Autodesk Fusion 360 part; units mm, degrees
note: some values were not read from the file. Set by a fixed rule: which sketch regions a step uses.
(part 2 of 10)
  spline S7 degree 5 poles (14.007, -3.8365) (14.007, -3.8365) (14.0072, -3.8366) (14.0074, -3.8366) (14.0077, -3.8367) (14.0083, -3.8369) (14.0089, -3.837) (14.0095, -3.8372) (14.0103, -3.8374) (14.0111, -3.8376) (14.012, -3.8378) (14.013, -3.838) (14.0141, -3.8383) (14.0152, -3.8386) (14.0164, -3.8388) (14.0177, -3.8391) (14.019, -3.8394) (14.0204, -3.8398) (14.0219, -3.8401) (14.0235, -3.8405) (14.0251, -3.8408) (14.0268, -3.8412) (14.0286, -3.8416) (14.0305, -3.842) (14.0324, -3.8424) (14.0343, -3.8428) (14.0364, -3.8432) (14.0385, -3.8436) (14.0407, -3.8441) (14.0429, -3.8445) (14.0452, -3.845) (14.0476, -3.8454) (14.05, -3.8459) (14.0525, -3.8464) (14.0551, -3.8469) (14.0577, -3.8473) (14.0604, -3.8478) (14.0632, -3.8483) (14.066, -3.8488) (14.0688, -3.8493) (14.0718, -3.8498) (14.0748, -3.8504) (14.0778, -3.8509) (14.0809, -3.8514) (14.0841, -3.8519) (14.0873, -3.8525) (14.0906, -3.853) (14.094, -3.8535) (14.0974, -3.854) (14.1009, -3.8546) (14.1044, -3.8551) (14.1079, -3.8557) (14.1116, -3.8562) (14.1153, -3.8567) (14.119, -3.8573) (14.1228, -3.8578) (14.1267, -3.8583) (14.1306, -3.8589) (14.1345, -3.8594) (14.1386, -3.86) (14.1426, -3.8605) (14.1467, -3.861) (14.1509, -3.8615) (14.1552, -3.8621) (14.1594, -3.8626) (14.1638, -3.8631) (14.1682, -3.8636) (14.1726, -3.8642) (14.1771, -3.8647) (14.1816, -3.8652) (14.1862, -3.8657) (14.1908, -3.8662) (14.1955, -3.8667) (14.2003, -3.8672) (14.2051, -3.8677) (14.2099, -3.8682) (14.2148, -3.8686) (14.2197, -3.8691) (14.2247, -3.8696) (14.2297, -3.87) (14.2348, -3.8705) (14.2399, -3.871) (14.2451, -3.8714) (14.2503, -3.8718) (14.2556, -3.8723) (14.2609, -3.8727) (14.2663, -3.8731) (14.2717, -3.8735) (14.2771, -3.8739) (14.2826, -3.8743) (14.2882, -3.8747) (14.2938, -3.8751) (14.2994, -3.8755) (14.3051, -3.8758) (14.3108, -3.8762) (14.3166, -3.8766) (14.3224, -3.8769) (14.3283, -3.8772) (14.3342, -3.8776) (14.3401, -3.8779) (14.3461, -3.8782) (14.3521, -3.8785) (14.3582, -3.8788) (14.3643, -3.879) (14.3705, -3.8793) (14.3767, -3.8796) (14.3829, -3.8798) (14.3892, -3.88) (14.3955, -3.8803) (14.4019, -3.8805) (14.4083, -3.8807) (14.4147, -3.8809) (14.4212, -3.8811) (14.4277, -3.8812) (14.4343, -3.8814) (14.4409, -3.8816) (14.4476, -3.8817) (14.4542, -3.8818) (14.461, -3.8819) (14.4677, -3.882) (14.4745, -3.8821) (14.4814, -3.8822) (14.4883, -3.8823) (14.4952, -3.8823) (14.5021, -3.8824) (14.5091, -3.8824) (14.5162, -3.8824) (14.5233, -3.8824) (14.5304, -3.8824) (14.5375, -3.8824) (14.5447, -3.8824) (14.5519, -3.8823) (14.5592, -3.8823) (14.5665, -3.8822) (14.5738, -3.8821) (14.5812, -3.882) (14.5886, -3.8819) (14.596, -3.8817) (14.6035, -3.8816) (14.611, -3.8814) (14.6186, -3.8813) (14.6261, -3.8811) (14.6338, -3.8809) (14.6414, -3.8807) (14.6491, -3.8804) (14.6568, -3.8802) (14.6646, -3.8799) (14.6724, -3.8797) (14.6802, -3.8794) (14.6881, -3.8791) (14.696, -3.8787) (14.7039, -3.8784) (14.7119, -3.878) (14.7199, -3.8777) (14.7279, -3.8773) (14.7359, -3.8769) (14.744, -3.8765) (14.7522, -3.8761) (14.7603, -3.8756) (14.7685, -3.8751) (14.7768, -3.8747) (14.785, -3.8742) (14.7933, -3.8737) (14.8016, -3.8731) (14.81, -3.8726) (14.8184, -3.872) (14.8268, -3.8714) (14.8352, -3.8708) (14.8437, -3.8702) (14.8522, -3.8696) (14.8608, -3.869) (14.8693, -3.8683) (14.8779, -3.8676) (14.8866, -3.8669) (14.8952, -3.8662) (14.9039, -3.8655) (14.9127, -3.8647) (14.9214, -3.8639) (14.9302, -3.8632) (14.939, -3.8624) (14.9479, -3.8615) (14.9567, -3.8607) (14.9656, -3.8598) (14.9746, -3.859) (14.9835, -3.8581) (14.9925, -3.8572) (15.0015, -3.8562) (15.0106, -3.8553) (15.0197, -3.8543) (15.0288, -3.8533) (15.0379, -3.8523) (15.0471, -3.8513) (15.0563, -3.8503) (15.0655, -3.8492) (15.0747, -3.8481) (15.084, -3.847) (15.0933, -3.8459) (15.1026, -3.8448) (15.112, -3.8436) (15.1214, -3.8424) (15.1308, -3.8412) (15.1402, -3.84) (15.1497, -3.8388) (15.1591, -3.8375) (15.1687, -3.8363) (15.1782, -3.835) (15.1878, -3.8337) (15.1974, -3.8323) (15.207, -3.831) (15.2166, -3.8296) (15.2263, -3.8282) (15.236, -3.8268) (15.2457, -3.8254) (15.2555, -3.8239) (15.2653, -3.8225) (15.2751, -3.821) (15.2849, -3.8195) (15.2947, -3.8179) (15.3046, -3.8164) (15.3145, -3.8148) (15.3244, -3.8132) (15.3344, -3.8116) (15.3444, -3.81) (15.3544, -3.8083) (15.3644, -3.8067) (15.3744, -3.805) (15.3845, -3.8033) (15.3946, -3.8015) (15.4047, -3.7998) (15.4148, -3.798) (15.425, -3.7962) (15.4352, -3.7944) (15.4454, -3.7925) (15.4556, -3.7907) (15.4659, -3.7888) (15.4762, -3.7869) (15.4865, -3.7849) (15.4968, -3.783) (15.5072, -3.781) (15.5175, -3.779) (15.5279, -3.777) (15.5363, -3.7754) (15.5425, -3.7742) (15.5467, -3.7733) (15.5488, -3.7729) knots 0 0 0 0 0 0 0.00416667 0.00833333 0.0125 0.01666667 0.02083333 0.025 0.02916667 0.03333333 0.0375 0.04166667 0.04583333 0.05 0.05416667 0.05833333 0.0625 0.06666667 0.07083333 0.075 0.07916667 0.08333333 0.0875 0.09166667 0.09583333 0.1 0.10416667 0.10833333 0.1125 0.11666667 0.12083333 0.125 0.12916667 0.13333333 0.1375 0.14166667 0.14583333 0.15 0.15416667 0.15833333 0.1625 0.16666667 0.17083333 0.175 0.17916667 0.18333333 0.1875 0.19166667 0.19583333 0.2 0.20416667 0.20833333 0.2125 0.21666667 0.22083333 0.225 0.22916667 0.23333333 0.2375 0.24166667 0.24583333 0.25 0.25416667 0.25833333 0.2625 0.26666667 0.27083333 0.275 0.27916667 0.28333333 0.2875 0.29166667 0.29583333 0.3 0.30416667 0.30833333 0.3125 0.31666667 0.32083333 0.325 0.32916667 0.33333333 0.3375 0.34166667 0.34583333 0.35 0.35416667 0.35833333 0.3625 0.36666667 0.37083333 0.375 0.37916667 0.38333333 0.3875 0.39166667 0.39583333 0.4 0.40416667 0.40833333 0.4125 0.41666667 0.42083333 0.425 0.42916667 0.43333333 0.4375 0.44166667 0.44583333 0.45 0.45416667 0.45833333 0.4625 0.46666667 0.47083333 0.475 0.47916667 0.48333333 0.4875 0.49166667 0.49583333 0.5 0.50416667 0.50833333 0.5125 0.51666667 0.52083333 0.525 0.52916667 0.53333333 0.5375 0.54166667 0.54583333 0.55 0.55416667 0.55833333 0.5625 0.56666667 0.57083333 0.575 0.57916667 0.58333333 0.5875 0.59166667 0.59583333 0.6 0.60416667 0.60833333 0.6125 0.61666667 0.62083333 0.625 0.62916667 0.63333333 0.6375 0.64166667 0.64583333 0.65 0.65416667 0.65833333 0.6625 0.66666667 0.67083333 0.675 0.67916667 0.68333333 0.6875 0.69166667 0.69583333 0.7 0.70416667 0.70833333 0.7125 0.71666667 0.72083333 0.725 0.72916667 0.73333333 0.7375 0.74166667 0.74583333 0.75 0.75416667 0.75833333 0.7625 0.76666667 0.77083333 0.775 0.77916667 0.78333333 0.7875 0.79166667 0.79583333 0.8 0.80416667 0.80833333 0.8125 0.81666667 0.82083333 0.825 0.82916667 0.83333333 0.8375 0.84166667 0.84583333 0.85 0.85416667 0.85833333 0.8625 0.86666667 0.87083333 0.875 0.87916667 0.88333333 0.8875 0.89166667 0.89583333 0.9 0.90416667 0.90833333 0.9125 0.91666667 0.92083333 0.925 0.92916667 0.93333333 0.9375 0.94166667 0.94583333 0.95 0.95416667 0.95833333 0.9625 0.96666667 0.97083333 0.975 0.97916667 0.98333333 0.9875 0.99166667 0.99583333 1 1 1 1 1 1
  arc A6 (15.5488, -3.7729) -> (15.7391, -2.8775) centre (0, 0) ccw
  line L7 (12.9032, 6.6649) -> (12.9026, 6.6646)
  line L8 (13.5863, 5.129) -> (13.5869, 5.1293)
  arc A7 (14.7969, 6.087) -> (14.4246, 6.9233) centre (0, 0) ccw
  arc A8 (15.7391, 2.8775) -> (15.5488, 3.7729) centre (0, 0) ccw
  line L9 (12.8639, 4.8563) -> (13.5863, 5.129)
  circle A9 centre (-7.0711, -7.0711) radius 1.7
  spline S8 degree 5 poles (14.4985, -0.8405) (14.4986, -0.8405) (14.4987, -0.8405) (14.499, -0.8405) (14.4993, -0.8405) (14.4999, -0.8405) (14.5005, -0.8406) (14.5012, -0.8406) (14.502, -0.8406) (14.5028, -0.8406) (14.5037, -0.8407) (14.5048, -0.8407) (14.5058, -0.8407) (14.507, -0.8407) (14.5082, -0.8408) (14.5096, -0.8408) (14.5109, -0.8408) (14.5124, -0.8408) (14.5139, -0.8409) (14.5155, -0.8409) (14.5172, -0.8409) (14.519, -0.8409) (14.5208, -0.8409) (14.5226, -0.8409) (14.5246, -0.8409) (14.5266, -0.8409) (14.5287, -0.8409) (14.5309, -0.8409) (14.5331, -0.8408) (14.5354, -0.8408) (14.5377, -0.8408) (14.5401, -0.8407) (14.5426, -0.8407) (14.5452, -0.8406) (14.5478, -0.8406) (14.5504, -0.8405) (14.5532, -0.8404) (14.556, -0.8403) (14.5588, -0.8402) (14.5617, -0.8401) (14.5647, -0.84) (14.5677, -0.8399) (14.5708, -0.8398) (14.574, -0.8396) (14.5772, -0.8395) (14.5805, -0.8393) (14.5838, -0.8392) (14.5872, -0.839) (14.5906, -0.8388) (14.5941, -0.8386) (14.5977, -0.8384) (14.6013, -0.8382) (14.605, -0.838) (14.6087, -0.8377) (14.6124, -0.8375) (14.6163, -0.8372) (14.6202, -0.8369) (14.6241, -0.8366) (14.6281, -0.8363) (14.6321, -0.836) (14.6362, -0.8357) (14.6404, -0.8354) (14.6446, -0.835) (14.6488, -0.8347) (14.6531, -0.8343) (14.6574, -0.8339) (14.6618, -0.8335) (14.6663, -0.8331) (14.6708, -0.8326) (14.6753, -0.8322) (14.6799, -0.8317) (14.6846, -0.8313) (14.6893, -0.8308) (14.694, -0.8303) (14.6988, -0.8298) (14.7036, -0.8292) (14.7085, -0.8287) (14.7134, -0.8281) (14.7184, -0.8275) (14.7234, -0.8269) (14.7285, -0.8263) (14.7336, -0.8257) (14.7387, -0.8251) (14.7439, -0.8244) (14.7492, -0.8237) (14.7545, -0.8231) (14.7598, -0.8224) (14.7652, -0.8216) (14.7706, -0.8209) (14.7761, -0.8201) (14.7816, -0.8194) (14.7871, -0.8186) (14.7927, -0.8178) (14.7983, -0.817) (14.804, -0.8161) (14.8097, -0.8153) (14.8155, -0.8144) (14.8213, -0.8135) (14.8271, -0.8126) (14.833, -0.8117) (14.8389, -0.8107) (14.8449, -0.8097) (14.8509, -0.8088) (14.8569, -0.8078) (14.863, -0.8067) (14.8691, -0.8057) (14.8753, -0.8047) (14.8814, -0.8036) (14.8877, -0.8025) (14.8939, -0.8014) (14.9003, -0.8002) (14.9066, -0.7991) (14.913, -0.7979) (14.9194, -0.7967) (14.9259, -0.7955) (14.9324, -0.7943) (14.9389, -0.7931) (14.9455, -0.7918) (14.9521, -0.7905) (14.9587, -0.7892) (14.9654, -0.7879) (14.9721, -0.7865) (14.9788, -0.7852) (14.9856, -0.7838) (14.9924, -0.7824) (14.9993, -0.781) (15.0062, -0.7795) (15.0131, -0.778) (15.02, -0.7766) (15.027, -0.775) (15.0341, -0.7735) (15.0411, -0.772) (15.0482, -0.7704) (15.0553, -0.7688) (15.0625, -0.7672) (15.0697, -0.7656) (15.0769, -0.7639) (15.0841, -0.7622) (15.0914, -0.7605) (15.0987, -0.7588) (15.1061, -0.7571) (15.1135, -0.7553) (15.1209, -0.7535) (15.1283, -0.7517) (15.1358, -0.7499) (15.1433, -0.7481) (15.1508, -0.7462) (15.1584, -0.7443) (15.166, -0.7424) (15.1736, -0.7405) (15.1813, -0.7385) (15.1889, -0.7365) (15.1967, -0.7345) (15.2044, -0.7325) (15.2122, -0.7305) (15.22, -0.7284) (15.2278, -0.7263) (15.2357, -0.7242) (15.2436, -0.7221) (15.2515, -0.7199) (15.2594, -0.7177) (15.2674, -0.7155) (15.2754, -0.7133) (15.2834, -0.7111) (15.2915, -0.7088) (15.2996, -0.7065) (15.3077, -0.7042) (15.3158, -0.7018) (15.324, -0.6995) (15.3322, -0.6971) (15.3404, -0.6947) (15.3487, -0.6923) (15.3569, -0.6898) (15.3652, -0.6873) (15.3736, -0.6848) (15.3819, -0.6823) (15.3903, -0.6797) (15.3987, -0.6772) (15.4071, -0.6746) (15.4156, -0.672) (15.4241, -0.6693) (15.4326, -0.6667) (15.4411, -0.664) (15.4497, -0.6613) (15.4582, -0.6585) (15.4668, -0.6558) (15.4755, -0.653) (15.4841, -0.6502) (15.4928, -0.6473) (15.5015, -0.6445) (15.5102, -0.6416) (15.519, -0.6387) (15.5278, -0.6358) (15.5365, -0.6328) (15.5454, -0.6298) (15.5542, -0.6268) (15.5631, -0.6238) (15.572, -0.6207) (15.5809, -0.6177) (15.5898, -0.6146) (15.5988, -0.6114) (15.6077, -0.6083) (15.6167, -0.6051) (15.6258, -0.6019) (15.6348, -0.5987) (15.6439, -0.5955) (15.653, -0.5922) (15.6621, -0.5889) (15.6712, -0.5856) (15.6803, -0.5822) (15.6895, -0.5789) (15.6987, -0.5755) (15.7079, -0.572) (15.7172, -0.5686) (15.7264, -0.5651) (15.7357, -0.5616) (15.745, -0.5581) (15.7543, -0.5546) (15.7636, -0.551) (15.773, -0.5474) (15.7824, -0.5438) (15.7918, -0.5401) (15.8012, -0.5365) (15.8106, -0.5328) (15.8201, -0.529) (15.8295, -0.5253) (15.839, -0.5215) (15.8486, -0.5177) (15.8581, -0.5139) (15.8676, -0.5101) (15.8772, -0.5062) (15.8868, -0.5023) (15.8964, -0.4984) (15.906, -0.4944) (15.9157, -0.4904) (15.9253, -0.4864) (15.935, -0.4824) (15.9447, -0.4784) (15.9544, -0.4743) (15.9641, -0.4702) (15.9739, -0.466) (15.9817, -0.4627) (15.9876, -0.4602) (15.9915, -0.4585) (15.9935, -0.4577) knots 0 0 0 0 0 0 0.00416667 0.00833333 0.0125 0.01666667 0.02083333 0.025 0.02916667 0.03333333 0.0375 0.04166667 0.04583333 0.05 0.05416667 0.05833333 0.0625 0.06666667 0.07083333 0.075 0.07916667 0.08333333 0.0875 0.09166667 0.09583333 0.1 0.10416667 0.10833333 0.1125 0.11666667 0.12083333 0.125 0.12916667 0.13333333 0.1375 0.14166667 0.14583333 0.15 0.15416667 0.15833333 0.1625 0.16666667 0.17083333 0.175 0.17916667 0.18333333 0.1875 0.19166667 0.19583333 0.2 0.20416667 0.20833333 0.2125 0.21666667 0.22083333 0.225 0.22916667 0.23333333 0.2375 0.24166667 0.24583333 0.25 0.25416667 0.25833333 0.2625 0.26666667 0.27083333 0.275 0.27916667 0.28333333 0.2875 0.29166667 0.29583333 0.3 0.30416667 0.30833333 0.3125 0.31666667 0.32083333 0.325 0.32916667 0.33333333 0.3375 0.34166667 0.34583333 0.35 0.35416667 0.35833333 0.3625 0.36666667 0.37083333 0.375 0.37916667 0.38333333 0.3875 0.39166667 0.39583333 0.4 0.40416667 0.40833333 0.4125 0.41666667 0.42083333 0.425 0.42916667 0.43333333 0.4375 0.44166667 0.44583333 0.45 0.45416667 0.45833333 0.4625 0.46666667 0.47083333 0.475 0.47916667 0.48333333 0.4875 0.49166667 0.49583333 0.5 0.50416667 0.50833333 0.5125 0.51666667 0.52083333 0.525 0.52916667 0.53333333 0.5375 0.54166667 0.54583333 0.55 0.55416667 0.55833333 0.5625 0.56666667 0.57083333 0.575 0.57916667 0.58333333 0.5875 0.59166667 0.59583333 0.6 0.60416667 0.60833333 0.6125 0.61666667 0.62083333 0.625 0.62916667 0.63333333 0.6375 0.64166667 0.64583333 0.65 0.65416667 0.65833333 0.6625 0.66666667 0.67083333 0.675 0.67916667 0.68333333 0.6875 0.69166667 0.69583333 0.7 0.70416667 0.70833333 0.7125 0.71666667 0.72083333 0.725 0.72916667 0.73333333 0.7375 0.74166667 0.74583333 0.75 0.75416667 0.75833333 0.7625 0.76666667 0.77083333 0.775 0.77916667 0.78333333 0.7875 0.79166667 0.79583333 0.8 0.80416667 0.80833333 0.8125 0.81666667 0.82083333 0.825 0.82916667 0.83333333 0.8375 0.84166667 0.84583333 0.85 0.85416667 0.85833333 0.8625 0.86666667 0.87083333 0.875 0.87916667 0.88333333 0.8875 0.89166667 0.89583333 0.9 0.90416667 0.90833333 0.9125 0.91666667 0.92083333 0.925 0.92916667 0.93333333 0.9375 0.94166667 0.94583333 0.95 0.95416667 0.95833333 0.9625 0.96666667 0.97083333 0.975 0.97916667 0.98333333 0.9875 0.99166667 0.99583333 1 1 1 1 1 1
  arc A10 (13.727, 0.7957) -> (13.5924, 2.0756) centre (0, 0) ccw
  arc A11 (15.9935, -0.4577) -> (15.9935, 0.4577) centre (0, 0) ccw
  spline S9 degree 5 poles (15.7391, -2.8775) (15.7374, -2.8763) (15.7339, -2.8738) (15.7287, -2.8702) (15.7217, -2.8653) (15.713, -2.8592) (15.7044, -2.8532) (15.6957, -2.8472) (15.6871, -2.8412) (15.6785, -2.8353) (15.6698, -2.8293) (15.6612, -2.8234) (15.6526, -2.8176) (15.6441, -2.8117) (15.6355, -2.8059) (15.6269, -2.8002) (15.6184, -2.7944) (15.6099, -2.7887) (15.6014, -2.783) (15.5929, -2.7773) (15.5844, -2.7717) (15.5759, -2.7661) (15.5674, -2.7605) (15.559, -2.755) (15.5505, -2.7494) (15.5421, -2.744) (15.5337, -2.7385) (15.5253, -2.7331) (15.517, -2.7277) (15.5086, -2.7223) (15.5002, -2.7169) (15.4919, -2.7116) (15.4836, -2.7063) (15.4753, -2.7011) (15.467, -2.6958) (15.4587, -2.6906) (15.4505, -2.6855) (15.4422, -2.6803) (15.434, -2.6752) (15.4258, -2.6701) (15.4176, -2.665) (15.4094, -2.66) (15.4013, -2.655) (15.3931, -2.65) (15.385, -2.6451) (15.3769, -2.6402) (15.3688, -2.6353) (15.3607, -2.6304) (15.3527, -2.6256) (15.3446, -2.6208) (15.3366, -2.616) (15.3286, -2.6113) (15.3206, -2.6065) (15.3126, -2.6019) (15.3047, -2.5972) (15.2968, -2.5926) (15.2888, -2.588) (15.2809, -2.5834) (15.2731, -2.5788) (15.2652, -2.5743) (15.2574, -2.5698) (15.2495, -2.5654) (15.2417, -2.5609) (15.2339, -2.5565) (15.2262, -2.5522) (15.2184, -2.5478) (15.2107, -2.5435) (15.203, -2.5392) (15.1953, -2.5349) (15.1876, -2.5307) (15.18, -2.5265) (15.1724, -2.5223) (15.1648, -2.5182) (15.1572, -2.514) (15.1496, -2.5099) (15.1421, -2.5059) (15.1346, -2.5018) (15.1271, -2.4978) (15.1196, -2.4939) (15.1121, -2.4899) (15.1047, -2.486) (15.0973, -2.4821) (15.0899, -2.4782) (15.0825, -2.4744) (15.0752, -2.4706) (15.0679, -2.4668) (15.0606, -2.463) (15.0533, -2.4593) (15.0461, -2.4556) (15.0388, -2.4519) (15.0316, -2.4483) (15.0245, -2.4447) (15.0173, -2.4411) (15.0102, -2.4375) (15.0031, -2.434) (14.996, -2.4305) (14.9889, -2.427) (14.9819, -2.4236) (14.9749, -2.4201) (14.9679, -2.4167) (14.9609, -2.4134) (14.954, -2.41) (14.9471, -2.4067) (14.9402, -2.4034) (14.9334, -2.4002) (14.9266, -2.397) (14.9198, -2.3938) (14.913, -2.3906) (14.9062, -2.3874) (14.8995, -2.3843) (14.8928, -2.3812) (14.8862, -2.3782) (14.8795, -2.3751) (14.8729, -2.3721) (14.8663, -2.3691) (14.8598, -2.3662) (14.8533, -2.3633) (14.8468, -2.3604) (14.8403, -2.3575) (14.8339, -2.3546) (14.8275, -2.3518) (14.8211, -2.349) (14.8148, -2.3463) (14.8084, -2.3435) (14.8022, -2.3408) (14.7959, -2.3381) (14.7897, -2.3355) (14.7835, -2.3328) (14.7773, -2.3302) (14.7712, -2.3277) (14.7651, -2.3251) (14.759, -2.3226) (14.753, -2.3201) (14.747, -2.3176) (14.741, -2.3152) (14.7351, -2.3128) (14.7292, -2.3104) (14.7233, -2.308) (14.7175, -2.3057) (14.7117, -2.3034) (14.7059, -2.3011) (14.7002, -2.2988) (14.6945, -2.2966) (14.6888, -2.2944) (14.6832, -2.2922) (14.6776, -2.29) (14.672, -2.2879) (14.6665, -2.2858) (14.661, -2.2837) (14.6556, -2.2817) (14.6502, -2.2796) (14.6448, -2.2776) (14.6395, -2.2757) (14.6342, -2.2737) (14.6289, -2.2718) (14.6237, -2.2699) (14.6185, -2.268) (14.6133, -2.2662) (14.6082, -2.2644) (14.6032, -2.2626) (14.5981, -2.2608) (14.5932, -2.259) (14.5882, -2.2573) (14.5833, -2.2556) (14.5784, -2.2539) (14.5736, -2.2523) (14.5688, -2.2507) (14.5641, -2.2491) (14.5594, -2.2475) (14.5547, -2.2459) (14.5501, -2.2444) (14.5455, -2.2429) (14.541, -2.2414) (14.5365, -2.24) (14.5321, -2.2386) (14.5277, -2.2372) (14.5233, -2.2358) (14.519, -2.2344) (14.5147, -2.2331) (14.5105, -2.2318) (14.5063, -2.2305) (14.5022, -2.2292) (14.4981, -2.228) (14.4941, -2.2268) (14.4901, -2.2256) (14.4862, -2.2244) (14.4823, -2.2233) (14.4785, -2.2222) (14.4747, -2.2211) (14.4709, -2.22) (14.4673, -2.2189) (14.4636, -2.2179) (14.46, -2.2169) (14.4565, -2.2159) (14.453, -2.2149) (14.4496, -2.214) (14.4462, -2.2131) (14.4429, -2.2122) (14.4396, -2.2113) (14.4364, -2.2104) (14.4332, -2.2096) (14.4301, -2.2088) (14.427, -2.208) (14.424, -2.2072) (14.4211, -2.2065) (14.4182, -2.2058) (14.4154, -2.2051) (14.4126, -2.2044) (14.4099, -2.2037) (14.4072, -2.2031) (14.4046, -2.2025) (14.4021, -2.2018) (14.3996, -2.2013) (14.3972, -2.2007) (14.3948, -2.2002) (14.3925, -2.1996) (14.3903, -2.1991) (14.3882, -2.1986) (14.386, -2.1982) (14.384, -2.1977) (14.382, -2.1973) (14.3801, -2.1969) (14.3783, -2.1965) (14.3765, -2.1961) (14.3748, -2.1958) (14.3732, -2.1954) (14.3716, -2.1951) (14.3701, -2.1948) (14.3687, -2.1945) (14.3673, -2.1943) (14.366, -2.194) (14.3648, -2.1938) (14.3637, -2.1936) (14.3626, -2.1934) (14.3616, -2.1932) (14.3607, -2.193) (14.3598, -2.1929) (14.3591, -2.1928) (14.3584, -2.1926) (14.3578, -2.1925) (14.3572, -2.1924) (14.3569, -2.1924) (14.3566, -2.1923) (14.3565, -2.1923) (14.3564, -2.1923) knots -1 -1 -1 -1 -1 -1 -0.99583333 -0.99166667 -0.9875 -0.98333333 -0.97916667 -0.975 -0.97083333 -0.96666667 -0.9625 -0.95833333 -0.95416667 -0.95 -0.94583333 -0.94166667 -0.9375 -0.93333333 -0.92916667 -0.925 -0.92083333 -0.91666667 -0.9125 -0.90833333 -0.90416667 -0.9 -0.89583333 -0.89166667 -0.8875 -0.88333333 -0.87916667 -0.875 -0.87083333 -0.86666667 -0.8625 -0.85833333 -0.85416667 -0.85 -0.84583333 -0.84166667 -0.8375 -0.83333333 -0.82916667 -0.825 -0.82083333 -0.81666667 -0.8125 -0.80833333 -0.80416667 -0.8 -0.79583333 -0.79166667 -0.7875 -0.78333333 -0.77916667 -0.775 -0.77083333 -0.76666667 -0.7625 -0.75833333 -0.75416667 -0.75 -0.74583333 -0.74166667 -0.7375 -0.73333333 -0.72916667 -0.725 -0.72083333 -0.71666667 -0.7125 -0.70833333 -0.70416667 -0.7 -0.69583333 -0.69166667 -0.6875 -0.68333333 -0.67916667 -0.675 -0.67083333 -0.66666667 -0.6625 -0.65833333 -0.65416667 -0.65 -0.64583333 -0.64166667 -0.6375 -0.63333333 -0.62916667 -0.625 -0.62083333 -0.61666667 -0.6125 -0.60833333 -0.60416667 -0.6 -0.59583333 -0.59166667 -0.5875 -0.58333333 -0.57916667 -0.575 -0.57083333 -0.56666667 -0.5625 -0.55833333 -0.55416667 -0.55 -0.54583333 -0.54166667 -0.5375 -0.53333333 -0.52916667 -0.525 -0.52083333 -0.51666667 -0.5125 -0.50833333 -0.50416667 -0.5 -0.49583333 -0.49166667 -0.4875 -0.48333333 -0.47916667 -0.475 -0.47083333 -0.46666667 -0.4625 -0.45833333 -0.45416667 -0.45 -0.44583333 -0.44166667 -0.4375 -0.43333333 -0.42916667 -0.425 -0.42083333 -0.41666667 -0.4125 -0.40833333 -0.40416667 -0.4 -0.39583333 -0.39166667 -0.3875 -0.38333333 -0.37916667 -0.375 -0.37083333 -0.36666667 -0.3625 -0.35833333 -0.35416667 -0.35 -0.34583333 -0.34166667 -0.3375 -0.33333333 -0.32916667 -0.325 -0.32083333 -0.31666667 -0.3125 -0.30833333 -0.30416667 -0.3 -0.29583333 -0.29166667 -0.2875 -0.28333333 -0.27916667 -0.275 -0.27083333 -0.26666667 -0.2625 -0.25833333 -0.25416667 -0.25 -0.24583333 -0.24166667 -0.2375 -0.23333333 -0.22916667 -0.225 -0.22083333 -0.21666667 -0.2125 -0.20833333 -0.20416667 -0.2 -0.19583333 -0.19166667 -0.1875 -0.18333333 -0.17916667 -0.175 -0.17083333 -0.16666667 -0.1625 -0.15833333 -0.15416667 -0.15 -0.14583333 -0.14166667 -0.1375 -0.13333333 -0.12916667 -0.125 -0.12083333 -0.11666667 -0.1125 -0.10833333 -0.10416667 -0.1 -0.09583333 -0.09166667 -0.0875 -0.08333333 -0.07916667 -0.075 -0.07083333 -0.06666667 -0.0625 -0.05833333 -0.05416667 -0.05 -0.04583333 -0.04166667 -0.0375 -0.03333333 -0.02916667 -0.025 -0.02083333 -0.01666667 -0.0125 -0.00833333 -0.00416667 0 0 0 0 0 0
  line L10 (14.0063, 3.8363) -> (13.2615, 3.6324)
  line L11 (-13.5863, -5.129) -> (-13.5869, -5.1293)
  circle A12 centre (10, 0) radius 1.7
  line L12 (-12.8639, -4.8563) -> (-13.5863, -5.129)
  line L13 (14.007, 3.8365) -> (14.0063, 3.8363)
  line L14 (-12.9032, -6.6649) -> (-12.9026, -6.6646)
  circle A13 centre (7.0711, -7.0711) radius 1.7
  line L15 (-11.2355, -9.202) -> (-11.235, -9.2016)
  line L16 (12.2236, -7.8421) -> (12.223, -7.8417)
  line L17 (12.223, -7.8417) -> (11.5731, -7.4247)
  line L18 (12.2165, -6.3102) -> (12.9026, -6.6646)
  line L19 (12.9026, -6.6646) -> (12.9032, -6.6649)
  arc A14 (-7.5526, 11.49) -> (-8.5938, 10.7336) centre (0, 0) ccw
  spline S10 degree 5 poles (-6.5214, 12.9763) (-6.5214, 12.9764) (-6.5215, 12.9765) (-6.5216, 12.9767) (-6.5218, 12.977) (-6.522, 12.9775) (-6.5223, 12.9781) (-6.5226, 12.9787) (-6.523, 12.9794) (-6.5234, 12.9801) (-6.5238, 12.9809) (-6.5243, 12.9818) (-6.5248, 12.9828) (-6.5254, 12.9838) (-6.526, 12.9849) (-6.5266, 12.986) (-6.5273, 12.9873) (-6.528, 12.9885) (-6.5288, 12.9899) (-6.5295, 12.9913) (-6.5304, 12.9927) (-6.5312, 12.9942) (-6.5321, 12.9958) (-6.5331, 12.9974) (-6.5341, 12.9991) (-6.5351, 13.0009) (-6.5361, 13.0027) (-6.5372, 13.0045) (-6.5384, 13.0064) (-6.5395, 13.0084) (-6.5407, 13.0104) (-6.542, 13.0125) (-6.5433, 13.0146) (-6.5446, 13.0168) (-6.5459, 13.019) (-6.5473, 13.0213) (-6.5488, 13.0236) (-6.5502, 13.026) (-6.5517, 13.0284) (-6.5533, 13.0309) (-6.5549, 13.0334) (-6.5565, 13.036) (-6.5581, 13.0386) (-6.5598, 13.0413) (-6.5616, 13.044) (-6.5633, 13.0467) (-6.5651, 13.0495) (-6.567, 13.0524) (-6.5689, 13.0553) (-6.5708, 13.0582) (-6.5728, 13.0612) (-6.5747, 13.0642) (-6.5768, 13.0672) (-6.5788, 13.0703) (-6.581, 13.0735) (-6.5831, 13.0767) (-6.5853, 13.0799) (-6.5875, 13.0832) (-6.5897, 13.0865) (-6.592, 13.0898) (-6.5944, 13.0932) (-6.5967, 13.0966) (-6.5991, 13.1001) (-6.6016, 13.1036) (-6.604, 13.1071) (-6.6065, 13.1107) (-6.6091, 13.1143) (-6.6117, 13.1179) (-6.6143, 13.1216) (-6.617, 13.1253) (-6.6197, 13.1291) (-6.6224, 13.1328) (-6.6252, 13.1367) (-6.628, 13.1405) (-6.6308, 13.1444) (-6.6337, 13.1483) (-6.6366, 13.1523) (-6.6395, 13.1563) (-6.6425, 13.1603) (-6.6455, 13.1643) (-6.6486, 13.1684) (-6.6517, 13.1725) (-6.6548, 13.1767) (-6.658, 13.1808) (-6.6612, 13.185) (-6.6644, 13.1893) (-6.6677, 13.1935) (-6.671, 13.1978) (-6.6744, 13.2022) (-6.6778, 13.2065) (-6.6812, 13.2109) (-6.6846, 13.2153) (-6.6881, 13.2197) (-6.6917, 13.2242) (-6.6952, 13.2287) (-6.6988, 13.2332) (-6.7025, 13.2378) (-6.7061, 13.2423) (-6.7098, 13.2469) (-6.7136, 13.2516) (-6.7174, 13.2562) (-6.7212, 13.2609) (-6.725, 13.2656) (-6.7289, 13.2703) (-6.7328, 13.2751) (-6.7368, 13.2799) (-6.7408, 13.2847) (-6.7448, 13.2895) (-6.7489, 13.2944) (-6.753, 13.2992) (-6.7571, 13.3041) (-6.7613, 13.309) (-6.7655, 13.314) (-6.7697, 13.319) (-6.774, 13.3239) (-6.7783, 13.329) (-6.7826, 13.334) (-6.787, 13.339) (-6.7914, 13.3441) (-6.7959, 13.3492) (-6.8004, 13.3543) (-6.8049, 13.3595) (-6.8094, 13.3646) (-6.814, 13.3698) (-6.8187, 13.375) (-6.8233, 13.3802) (-6.828, 13.3855) (-6.8327, 13.3907) (-6.8375, 13.396) (-6.8423, 13.4013) (-6.8471, 13.4066) (-6.852, 13.412) (-6.8569, 13.4173) (-6.8618, 13.4227) (-6.8668, 13.4281) (-6.8718, 13.4335) (-6.8769, 13.4389) (-6.8819, 13.4444) (-6.8871, 13.4498) (-6.8922, 13.4553) (-6.8974, 13.4608) (-6.9026, 13.4663) (-6.9078, 13.4718) (-6.9131, 13.4774) (-6.9184, 13.4829) (-6.9238, 13.4885) (-6.9292, 13.4941) (-6.9346, 13.4997) (-6.94, 13.5053) (-6.9455, 13.511) (-6.9511, 13.5166) (-6.9566, 13.5223) (-6.9622, 13.528) (-6.9678, 13.5337) (-6.9735, 13.5394) (-6.9792, 13.5451) (-6.9849, 13.5508) (-6.9907, 13.5566) (-6.9965, 13.5624) (-7.0023, 13.5681) (-7.0081, 13.5739) (-7.014, 13.5797) (-7.02, 13.5855) (-7.0259, 13.5914) (-7.0319, 13.5972) (-7.0379, 13.6031) (-7.044, 13.6089) (-7.0501, 13.6148) (-7.0562, 13.6207) (-7.0624, 13.6266) (-7.0686, 13.6325) (-7.0748, 13.6385) (-7.0811, 13.6444) (-7.0874, 13.6504) (-7.0937, 13.6563) (-7.1001, 13.6623) (-7.1065, 13.6683) (-7.1129, 13.6743) (-7.1194, 13.6803) (-7.1259, 13.6863) (-7.1324, 13.6923) (-7.1389, 13.6983) (-7.1455, 13.7044) (-7.1522, 13.7104) (-7.1588, 13.7165) (-7.1655, 13.7226) (-7.1723, 13.7286) (-7.179, 13.7347) (-7.1858, 13.7408) (-7.1926, 13.7469) (-7.1995, 13.753) (-7.2064, 13.7592) (-7.2133, 13.7653) (-7.2203, 13.7714) (-7.2272, 13.7776) (-7.2343, 13.7837) (-7.2413, 13.7899) (-7.2484, 13.7961) (-7.2555, 13.8023) (-7.2627, 13.8084) (-7.2699, 13.8146) (-7.2771, 13.8208) (-7.2843, 13.827) (-7.2916, 13.8333) (-7.2989, 13.8395) (-7.3063, 13.8457) (-7.3136, 13.8519) (-7.321, 13.8582) (-7.3285, 13.8644) (-7.336, 13.8707) (-7.3435, 13.8769) (-7.351, 13.8832) (-7.3586, 13.8895) (-7.3662, 13.8958) (-7.3738, 13.902) (-7.3815, 13.9083) (-7.3892, 13.9146) (-7.3969, 13.9209) (-7.4046, 13.9272) (-7.4124, 13.9335) (-7.4203, 13.9398) (-7.4281, 13.9461) (-7.436, 13.9525) (-7.4439, 13.9588) (-7.4519, 13.9651) (-7.4599, 13.9714) (-7.4679, 13.9778) (-7.4759, 13.9841) (-7.484, 13.9905) (-7.4921, 13.9968) (-7.5002, 14.0032) (-7.5084, 14.0095) (-7.5166, 14.0159) (-7.5248, 14.0222) (-7.5331, 14.0286) (-7.5414, 14.035) (-7.5497, 14.0413) (-7.5581, 14.0477) (-7.5665, 14.0541) (-7.5749, 14.0604) (-7.5833, 14.0668) (-7.5901, 14.0719) (-7.5952, 14.0758) (-7.5986, 14.0783) (-7.6003, 14.0796) knots 0 0 0 0 0 0 0.00416667 0.00833333 0.0125 0.01666667 0.02083333 0.025 0.02916667 0.03333333 0.0375 0.04166667 0.04583333 0.05 0.05416667 0.05833333 0.0625 0.06666667 0.07083333 0.075 0.07916667 0.08333333 0.0875 0.09166667 0.09583333 0.1 0.10416667 0.10833333 0.1125 0.11666667 0.12083333 0.125 0.12916667 0.13333333 0.1375 0.14166667 0.14583333 0.15 0.15416667 0.15833333 0.1625 0.16666667 0.17083333 0.175 0.17916667 0.18333333 0.1875 0.19166667 0.19583333 0.2 0.20416667 0.20833333 0.2125 0.21666667 0.22083333 0.225 0.22916667 0.23333333 0.2375 0.24166667 0.24583333 0.25 0.25416667 0.25833333 0.2625 0.26666667 0.27083333 0.275 0.27916667 0.28333333 0.2875 0.29166667 0.29583333 0.3 0.30416667 0.30833333 0.3125 0.31666667 0.32083333 0.325 0.32916667 0.33333333 0.3375 0.34166667 0.34583333 0.35 0.35416667 0.35833333 0.3625 0.36666667 0.37083333 0.375 0.37916667 0.38333333 0.3875 0.39166667 0.39583333 0.4 0.40416667 0.40833333 0.4125 0.41666667 0.42083333 0.425 0.42916667 0.43333333 0.4375 0.44166667 0.44583333 0.45 0.45416667 0.45833333 0.4625 0.46666667 0.47083333 0.475 0.47916667 0.48333333 0.4875 0.49166667 0.49583333 0.5 0.50416667 0.50833333 0.5125 0.51666667 0.52083333 0.525 0.52916667 0.53333333 0.5375 0.54166667 0.54583333 0.55 0.55416667 0.55833333 0.5625 0.56666667 0.57083333 0.575 0.57916667 0.58333333 0.5875 0.59166667 0.59583333 0.6 0.60416667 0.60833333 0.6125 0.61666667 0.62083333 0.625 0.62916667 0.63333333 0.6375 0.64166667 0.64583333 0.65 0.65416667 0.65833333 0.6625 0.66666667 0.67083333 0.675 0.67916667 0.68333333 0.6875 0.69166667 0.69583333 0.7 0.70416667 0.70833333 0.7125 0.71666667 0.72083333 0.725 0.72916667 0.73333333 0.7375 0.74166667 0.74583333 0.75 0.75416667 0.75833333 0.7625 0.76666667 0.77083333 0.775 0.77916667 0.78333333 0.7875 0.79166667 0.79583333 0.8 0.80416667 0.80833333 0.8125 0.81666667 0.82083333 0.825 0.82916667 0.83333333 0.8375 0.84166667 0.84583333 0.85 0.85416667 0.85833333 0.8625 0.86666667 0.87083333 0.875 0.87916667 0.88333333 0.8875 0.89166667 0.89583333 0.9 0.90416667 0.90833333 0.9125 0.91666667 0.92083333 0.925 0.92916667 0.93333333 0.9375 0.94166667 0.94583333 0.95 0.95416667 0.95833333 0.9625 0.96666667 0.97083333 0.975 0.97916667 0.98333333 0.9875 0.99166667 0.99583333 1 1 1 1 1 1
  line L20 (-9.7765, -9.6687) -> (-10.3255, -10.2117)
  line L21 (-11.235, 9.2016) -> (-11.2355, 9.202)
  arc A15 (-10.6376, -8.7123) -> (-9.7765, -9.6687) centre (0, 0) ccw
  line L22 (-11.235, -9.2016) -> (-10.6376, -8.7123)
  line L23 (-9.0764, 11.3364) -> (-9.0768, 11.3369)
  line L24 (6.5214, 12.9763) -> (6.5211, 12.9757)
  spline S11 degree 5 poles (-11.2355, 9.202) (-11.2356, 9.202) (-11.2357, 9.2021) (-11.2359, 9.2022) (-11.2362, 9.2025) (-11.2366, 9.2028) (-11.2371, 9.2032) (-11.2376, 9.2036) (-11.2382, 9.2041) (-11.2389, 9.2046) (-11.2396, 9.2052) (-11.2404, 9.2058) (-11.2413, 9.2065) (-11.2422, 9.2072) (-11.2432, 9.2079) (-11.2443, 9.2087) (-11.2454, 9.2096) (-11.2465, 9.2104) (-11.2478, 9.2113) (-11.2491, 9.2123) (-11.2504, 9.2133) (-11.2518, 9.2143) (-11.2533, 9.2154) (-11.2548, 9.2165) (-11.2564, 9.2177) (-11.258, 9.2188) (-11.2597, 9.22) (-11.2615, 9.2213) (-11.2633, 9.2226) (-11.2651, 9.2239) (-11.2671, 9.2253) (-11.269, 9.2266) (-11.2711, 9.2281) (-11.2732, 9.2295) (-11.2753, 9.231) (-11.2775, 9.2325) (-11.2798, 9.2341) (-11.2821, 9.2356) (-11.2844, 9.2372) (-11.2869, 9.2389) (-11.2893, 9.2405) (-11.2919, 9.2422) (-11.2944, 9.2439) (-11.2971, 9.2457) (-11.2998, 9.2474) (-11.3025, 9.2492) (-11.3053, 9.2511) (-11.3081, 9.2529) (-11.311, 9.2548) (-11.314, 9.2567) (-11.317, 9.2586) (-11.32, 9.2605) (-11.3231, 9.2625) (-11.3263, 9.2645) (-11.3295, 9.2665) (-11.3327, 9.2685) (-11.336, 9.2706) (-11.3394, 9.2727) (-11.3428, 9.2748) (-11.3462, 9.2769) (-11.3497, 9.2791) (-11.3533, 9.2812) (-11.3569, 9.2834) (-11.3605, 9.2856) (-11.3642, 9.2878) (-11.368, 9.2901) (-11.3718, 9.2923) (-11.3756, 9.2946) (-11.3795, 9.2969) (-11.3834, 9.2992) (-11.3874, 9.3015) (-11.3915, 9.3039) (-11.3955, 9.3062) (-11.3997, 9.3086) (-11.4038, 9.311) (-11.4081, 9.3134) (-11.4123, 9.3158) (-11.4167, 9.3183) (-11.421, 9.3207) (-11.4254, 9.3232) (-11.4299, 9.3257) (-11.4344, 9.3282) (-11.4389, 9.3307) (-11.4435, 9.3332) (-11.4482, 9.3358) (-11.4528, 9.3383) (-11.4576, 9.3409) (-11.4623, 9.3435) (-11.4672, 9.3461) (-11.472, 9.3487) (-11.4769, 9.3513) (-11.4819, 9.3539) (-11.4869, 9.3565) (-11.4919, 9.3592) (-11.497, 9.3618) (-11.5021, 9.3645) (-11.5073, 9.3672) (-11.5125, 9.3699) (-11.5178, 9.3725) (-11.5231, 9.3753) (-11.5284, 9.378) (-11.5338, 9.3807) (-11.5392, 9.3834) (-11.5447, 9.3862) (-11.5502, 9.3889) (-11.5558, 9.3917) (-11.5614, 9.3944) (-11.567, 9.3972) (-11.5727, 9.4) (-11.5784, 9.4028) (-11.5842, 9.4056) (-11.59, 9.4084) (-11.5959, 9.4112) (-11.6017, 9.414) (-11.6077, 9.4168) (-11.6137, 9.4196) (-11.6197, 9.4225) (-11.6257, 9.4253) (-11.6318, 9.4281) (-11.638, 9.431) (-11.6441, 9.4338) (-11.6504, 9.4367) (-11.6566, 9.4396) (-11.6629, 9.4424) (-11.6693, 9.4453) (-11.6756, 9.4482) (-11.6821, 9.451) (-11.6885, 9.4539) (-11.695, 9.4568) (-11.7016, 9.4597) (-11.7081, 9.4626) (-11.7148, 9.4655) (-11.7214, 9.4684) (-11.7281, 9.4713) (-11.7348, 9.4742) (-11.7416, 9.4771) (-11.7484, 9.48) (-11.7553, 9.4829) (-11.7622, 9.4858) (-11.7691, 9.4887) (-11.7761, 9.4916) (-11.7831, 9.4945) (-11.7901, 9.4975) (-11.7972, 9.5004) (-11.8043, 9.5033) (-11.8115, 9.5062) (-11.8187, 9.5091) (-11.8259, 9.512) (-11.8332, 9.515) (-11.8405, 9.5179) (-11.8478, 9.5208) (-11.8552, 9.5237) (-11.8626, 9.5266) (-11.8701, 9.5295) (-11.8776, 9.5325) (-11.8851, 9.5354) (-11.8926, 9.5383) (-11.9002, 9.5412) (-11.9079, 9.5441) (-11.9156, 9.547) (-11.9233, 9.5499) (-11.931, 9.5528) (-11.9388, 9.5557) (-11.9466, 9.5586) (-11.9545, 9.5615) (-11.9624, 9.5644) (-11.9703, 9.5673) (-11.9782, 9.5702) (-11.9862, 9.5731) (-11.9943, 9.576) (-12.0023, 9.5789) (-12.0104, 9.5818) (-12.0186, 9.5846) (-12.0267, 9.5875) (-12.035, 9.5904) (-12.0432, 9.5933) (-12.0515, 9.5961) (-12.0598, 9.599) (-12.0681, 9.6018) (-12.0765, 9.6047) (-12.0849, 9.6075) (-12.0934, 9.6104) (-12.1018, 9.6132) (-12.1104, 9.616) (-12.1189, 9.6189) (-12.1275, 9.6217) (-12.1361, 9.6245) (-12.1448, 9.6273) (-12.1535, 9.6301) (-12.1622, 9.6329) (-12.1709, 9.6357) (-12.1797, 9.6385) (-12.1885, 9.6413) (-12.1974, 9.6441) (-12.2063, 9.6469) (-12.2152, 9.6496) (-12.2241, 9.6524) (-12.2331, 9.6552) (-12.2421, 9.6579) (-12.2512, 9.6607) (-12.2603, 9.6634) (-12.2694, 9.6661) (-12.2785, 9.6688) (-12.2877, 9.6716) (-12.2969, 9.6743) (-12.3062, 9.677) (-12.3154, 9.6797) (-12.3247, 9.6823) (-12.3341, 9.685) (-12.3434, 9.6877) (-12.3528, 9.6904) (-12.3623, 9.693) (-12.3717, 9.6957) (-12.3812, 9.6983) (-12.3908, 9.7009) (-12.4003, 9.7036) (-12.4099, 9.7062) (-12.4195, 9.7088) (-12.4292, 9.7114) (-12.4389, 9.714) (-12.4486, 9.7166) (-12.4583, 9.7191) (-12.4681, 9.7217) (-12.4779, 9.7243) (-12.4877, 9.7268) (-12.4976, 9.7293) (-12.5075, 9.7319) (-12.5174, 9.7344) (-12.5274, 9.7369) (-12.5374, 9.7394) (-12.5474, 9.7419) (-12.5574, 9.7444) (-12.5675, 9.7469) (-12.5776, 9.7493) (-12.5878, 9.7518) (-12.5979, 9.7542) (-12.6081, 9.7566) (-12.6184, 9.7591) (-12.6286, 9.7615) (-12.6389, 9.7639) (-12.6492, 9.7663) (-12.6575, 9.7682) (-12.6637, 9.7696) (-12.6679, 9.7705) (-12.6699, 9.771) knots 0 0 0 0 0 0 0.00416667 0.00833333 0.0125 0.01666667 0.02083333 0.025 0.02916667 0.03333333 0.0375 0.04166667 0.04583333 0.05 0.05416667 0.05833333 0.0625 0.06666667 0.07083333 0.075 0.07916667 0.08333333 0.0875 0.09166667 0.09583333 0.1 0.10416667 0.10833333 0.1125 0.11666667 0.12083333 0.125 0.12916667 0.13333333 0.1375 0.14166667 0.14583333 0.15 0.15416667 0.15833333 0.1625 0.16666667 0.17083333 0.175 0.17916667 0.18333333 0.1875 0.19166667 0.19583333 0.2 0.20416667 0.20833333 0.2125 0.21666667 0.22083333 0.225 0.22916667 0.23333333 0.2375 0.24166667 0.24583333 0.25 0.25416667 0.25833333 0.2625 0.26666667 0.27083333 0.275 0.27916667 0.28333333 0.2875 0.29166667 0.29583333 0.3 0.30416667 0.30833333 0.3125 0.31666667 0.32083333 0.325 0.32916667 0.33333333 0.3375 0.34166667 0.34583333 0.35 0.35416667 0.35833333 0.3625 0.36666667 0.37083333 0.375 0.37916667 0.38333333 0.3875 0.39166667 0.39583333 0.4 0.40416667 0.40833333 0.4125 0.41666667 0.42083333 0.425 0.42916667 0.43333333 0.4375 0.44166667 0.44583333 0.45 0.45416667 0.45833333 0.4625 0.46666667 0.47083333 0.475 0.47916667 0.48333333 0.4875 0.49166667 0.49583333 0.5 0.50416667 0.50833333 0.5125 0.51666667 0.52083333 0.525 0.52916667 0.53333333 0.5375 0.54166667 0.54583333 0.55 0.55416667 0.55833333 0.5625 0.56666667 0.57083333 0.575 0.57916667 0.58333333 0.5875 0.59166667 0.59583333 0.6 0.60416667 0.60833333 0.6125 0.61666667 0.62083333 0.625 0.62916667 0.63333333 0.6375 0.64166667 0.64583333 0.65 0.65416667 0.65833333 0.6625 0.66666667 0.67083333 0.675 0.67916667 0.68333333 0.6875 0.69166667 0.69583333 0.7 0.70416667 0.70833333 0.7125 0.71666667 0.72083333 0.725 0.72916667 0.73333333 0.7375 0.74166667 0.74583333 0.75 0.75416667 0.75833333 0.7625 0.76666667 0.77083333 0.775 0.77916667 0.78333333 0.7875 0.79166667 0.79583333 0.8 0.80416667 0.80833333 0.8125 0.81666667 0.82083333 0.825 0.82916667 0.83333333 0.8375 0.84166667 0.84583333 0.85 0.85416667 0.85833333 0.8625 0.86666667 0.87083333 0.875 0.87916667 0.88333333 0.8875 0.89166667 0.89583333 0.9 0.90416667 0.90833333 0.9125 0.91666667 0.92083333 0.925 0.92916667 0.93333333 0.9375 0.94166667 0.94583333 0.95 0.95416667 0.95833333 0.9625 0.96666667 0.97083333 0.975 0.97916667 0.98333333 0.9875 0.99166667 0.99583333 1 1 1 1 1 1
  spline S12 degree 5 poles (-11.0419, 11.5792) (-11.0412, 11.5772) (-11.0398, 11.5731) (-11.0377, 11.5671) (-11.035, 11.5591) (-11.0315, 11.5491) (-11.028, 11.5391) (-11.0246, 11.5291) (-11.0211, 11.5192) (-11.0176, 11.5093) (-11.0141, 11.4995) (-11.0106, 11.4897) (-11.0071, 11.4799) (-11.0036, 11.4701) (-11.0001, 11.4604) (-10.9966, 11.4507) (-10.993, 11.441) (-10.9895, 11.4313) (-10.986, 11.4217) (-10.9824, 11.4122) (-10.9789, 11.4026) (-10.9753, 11.3931) (-10.9717, 11.3836) (-10.9682, 11.3742) (-10.9646, 11.3647) (-10.961, 11.3553) (-10.9574, 11.346) (-10.9538, 11.3367) (-10.9502, 11.3274) (-10.9466, 11.3181) (-10.943, 11.3089) (-10.9394, 11.2997) (-10.9358, 11.2905) (-10.9321, 11.2814) (-10.9285, 11.2723) (-10.9249, 11.2632) (-10.9212, 11.2541) (-10.9176, 11.2451) (-10.9139, 11.2362) (-10.9103, 11.2272) (-10.9066, 11.2183) (-10.903, 11.2094) (-10.8993, 11.2006) (-10.8957, 11.1918) (-10.892, 11.183) (-10.8883, 11.1743) (-10.8847, 11.1655) (-10.881, 11.1569) (-10.8773, 11.1482) (-10.8736, 11.1396) (-10.8699, 11.131) (-10.8662, 11.1225) (-10.8625, 11.114) (-10.8589, 11.1055) (-10.8552, 11.097) (-10.8515, 11.0886) (-10.8478, 11.0803) (-10.8441, 11.0719) (-10.8404, 11.0636) (-10.8367, 11.0553) (-10.833, 11.0471) (-10.8292, 11.0389) (-10.8255, 11.0307) (-10.8218, 11.0226) (-10.8181, 11.0145) (-10.8144, 11.0064) (-10.8107, 10.9984) (-10.807, 10.9903) (-10.8033, 10.9824) (-10.7996, 10.9745) (-10.7958, 10.9666) (-10.7921, 10.9587) (-10.7884, 10.9509) (-10.7847, 10.9431) (-10.781, 10.9353) (-10.7773, 10.9276) (-10.7736, 10.9199) (-10.7699, 10.9123) (-10.7662, 10.9046) (-10.7625, 10.8971) (-10.7587, 10.8895) (-10.755, 10.882) (-10.7513, 10.8745) (-10.7476, 10.8671) (-10.7439, 10.8597) (-10.7402, 10.8523) (-10.7365, 10.845) (-10.7328, 10.8377) (-10.7292, 10.8305) (-10.7255, 10.8233) (-10.7218, 10.8161) (-10.7181, 10.8089) (-10.7144, 10.8018) (-10.7107, 10.7947) (-10.7071, 10.7877) (-10.7034, 10.7807) (-10.6997, 10.7738) (-10.6961, 10.7668) (-10.6924, 10.7599) (-10.6888, 10.7531) (-10.6851, 10.7463) (-10.6815, 10.7395) (-10.6778, 10.7328) (-10.6742, 10.7261) (-10.6706, 10.7194) (-10.6669, 10.7128) (-10.6633, 10.7062) (-10.6597, 10.6997) (-10.6561, 10.6931) (-10.6525, 10.6867) (-10.6489, 10.6802) (-10.6453, 10.6738) (-10.6417, 10.6675) (-10.6381, 10.6612) (-10.6346, 10.6549) (-10.631, 10.6487) (-10.6275, 10.6425) (-10.6239, 10.6363) (-10.6204, 10.6302) (-10.6168, 10.6241) (-10.6133, 10.618) (-10.6098, 10.612) (-10.6063, 10.6061) (-10.6028, 10.6001) (-10.5993, 10.5943) (-10.5958, 10.5884) (-10.5923, 10.5826) (-10.5889, 10.5768) (-10.5854, 10.5711) (-10.582, 10.5654) (-10.5785, 10.5598) (-10.5751, 10.5542) (-10.5717, 10.5486) (-10.5683, 10.5431) (-10.5649, 10.5376) (-10.5615, 10.5321) (-10.5582, 10.5267) (-10.5548, 10.5214) (-10.5515, 10.516) (-10.5481, 10.5108) (-10.5448, 10.5055) (-10.5415, 10.5003) (-10.5382, 10.4952) (-10.5349, 10.4901) (-10.5316, 10.485) (-10.5284, 10.48) (-10.5251, 10.475) (-10.5219, 10.47) (-10.5187, 10.4651) (-10.5155, 10.4603) (-10.5123, 10.4554) (-10.5091, 10.4507) (-10.506, 10.4459) (-10.5028, 10.4412) (-10.4997, 10.4366) (-10.4966, 10.432) (-10.4935, 10.4274) (-10.4904, 10.4229) (-10.4874, 10.4184) (-10.4843, 10.414) (-10.4813, 10.4096) (-10.4783, 10.4052) (-10.4753, 10.4009) (-10.4723, 10.3967) (-10.4694, 10.3925) (-10.4664, 10.3883) (-10.4635, 10.3842) (-10.4606, 10.3801) (-10.4577, 10.376) (-10.4549, 10.3721) (-10.452, 10.3681) (-10.4492, 10.3642) (-10.4464, 10.3603) (-10.4436, 10.3565) (-10.4409, 10.3528) (-10.4382, 10.349) (-10.4354, 10.3454) (-10.4328, 10.3417) (-10.4301, 10.3382) (-10.4274, 10.3346) (-10.4248, 10.3311) (-10.4222, 10.3277) (-10.4197, 10.3243) (-10.4171, 10.3209) (-10.4146, 10.3176) (-10.4121, 10.3144) (-10.4096, 10.3112) (-10.4072, 10.308) (-10.4048, 10.3049) (-10.4024, 10.3018) (-10.4, 10.2988) (-10.3977, 10.2958) (-10.3954, 10.2929) (-10.3931, 10.29) (-10.3908, 10.2872) (-10.3886, 10.2844) (-10.3864, 10.2817) (-10.3842, 10.279) (-10.3821, 10.2764) (-10.38, 10.2738) (-10.3779, 10.2712) (-10.3759, 10.2688) (-10.3739, 10.2663) (-10.3719, 10.2639) (-10.37, 10.2616) (-10.368, 10.2593) (-10.3662, 10.2571) (-10.3643, 10.2549) (-10.3625, 10.2528) (-10.3608, 10.2507) (-10.359, 10.2486) (-10.3573, 10.2467) (-10.3557, 10.2447) (-10.354, 10.2429) (-10.3525, 10.241) (-10.3509, 10.2393) (-10.3494, 10.2376) (-10.3479, 10.2359) (-10.3465, 10.2343) (-10.3451, 10.2327) (-10.3438, 10.2312) (-10.3425, 10.2298) (-10.3412, 10.2284) (-10.34, 10.227) (-10.3388, 10.2257) (-10.3377, 10.2245) (-10.3366, 10.2233) (-10.3356, 10.2222) (-10.3346, 10.2211) (-10.3336, 10.2201) (-10.3327, 10.2191) (-10.3319, 10.2182) (-10.3311, 10.2174) (-10.3303, 10.2166) (-10.3296, 10.2159) (-10.329, 10.2152) (-10.3284, 10.2146) (-10.3279, 10.214) (-10.3274, 10.2135) (-10.3269, 10.2131) (-10.3266, 10.2127) (-10.3263, 10.2124) (-10.3261, 10.2123) (-10.326, 10.2122) (-10.326, 10.2121) knots -1 -1 -1 -1 -1 -1 -0.99583333 -0.99166667 -0.9875 -0.98333333 -0.97916667 -0.975 -0.97083333 -0.96666667 -0.9625 -0.95833333 -0.95416667 -0.95 -0.94583333 -0.94166667 -0.9375 -0.93333333 -0.92916667 -0.925 -0.92083333 -0.91666667 -0.9125 -0.90833333 -0.90416667 -0.9 -0.89583333 -0.89166667 -0.8875 -0.88333333 -0.87916667 -0.875 -0.87083333 -0.86666667 -0.8625 -0.85833333 -0.85416667 -0.85 -0.84583333 -0.84166667 -0.8375 -0.83333333 -0.82916667 -0.825 -0.82083333 -0.81666667 -0.8125 -0.80833333 -0.80416667 -0.8 -0.79583333 -0.79166667 -0.7875 -0.78333333 -0.77916667 -0.775 -0.77083333 -0.76666667 -0.7625 -0.75833333 -0.75416667 -0.75 -0.74583333 -0.74166667 -0.7375 -0.73333333 -0.72916667 -0.725 -0.72083333 -0.71666667 -0.7125 -0.70833333 -0.70416667 -0.7 -0.69583333 -0.69166667 -0.6875 -0.68333333 -0.67916667 -0.675 -0.67083333 -0.66666667 -0.6625 -0.65833333 -0.65416667 -0.65 -0.64583333 -0.64166667 -0.6375 -0.63333333 -0.62916667 -0.625 -0.62083333 -0.61666667 -0.6125 -0.60833333 -0.60416667 -0.6 -0.59583333 -0.59166667 -0.5875 -0.58333333 -0.57916667 -0.575 -0.57083333 -0.56666667 -0.5625 -0.55833333 -0.55416667 -0.55 -0.54583333 -0.54166667 -0.5375 -0.53333333 -0.52916667 -0.525 -0.52083333 -0.51666667 -0.5125 -0.50833333 -0.50416667 -0.5 -0.49583333 -0.49166667 -0.4875 -0.48333333 -0.47916667 -0.475 -0.47083333 -0.46666667 -0.4625 -0.45833333 -0.45416667 -0.45 -0.44583333 -0.44166667 -0.4375 -0.43333333 -0.42916667 -0.425 -0.42083333 -0.41666667 -0.4125 -0.40833333 -0.40416667 -0.4 -0.39583333 -0.39166667 -0.3875 -0.38333333 -0.37916667 -0.375 -0.37083333 -0.36666667 -0.3625 -0.35833333 -0.35416667 -0.35 -0.34583333 -0.34166667 -0.3375 -0.33333333 -0.32916667 -0.325 -0.32083333 -0.31666667 -0.3125 -0.30833333 -0.30416667 -0.3 -0.29583333 -0.29166667 -0.2875 -0.28333333 -0.27916667 -0.275 -0.27083333 -0.26666667 -0.2625 -0.25833333 -0.25416667 -0.25 -0.24583333 -0.24166667 -0.2375 -0.23333333 -0.22916667 -0.225 -0.22083333 -0.21666667 -0.2125 -0.20833333 -0.20416667 -0.2 -0.19583333 -0.19166667 -0.1875 -0.18333333 -0.17916667 -0.175 -0.17083333 -0.16666667 -0.1625 -0.15833333 -0.15416667 -0.15 -0.14583333 -0.14166667 -0.1375 -0.13333333 -0.12916667 -0.125 -0.12083333 -0.11666667 -0.1125 -0.10833333 -0.10416667 -0.1 -0.09583333 -0.09166667 -0.0875 -0.08333333 -0.07916667 -0.075 -0.07083333 -0.06666667 -0.0625 -0.05833333 -0.05416667 -0.05 -0.04583333 -0.04166667 -0.0375 -0.03333333 -0.02916667 -0.025 -0.02083333 -0.01666667 -0.0125 -0.00833333 -0.00416667 0 0 0 0 0 0
  line L25 (4.9987, 12.8092) -> (5.2794, 13.5286)
  arc A16 (-7.6003, 14.0796) -> (-8.3931, 13.6219) centre (0, 0) ccw
  arc A17 (-11.0419, -11.5792) -> (-10.3616, -12.1917) centre (0, 0) ccw
  line L26 (-7.9768, -12.1353) -> (-7.9771, -12.1359)